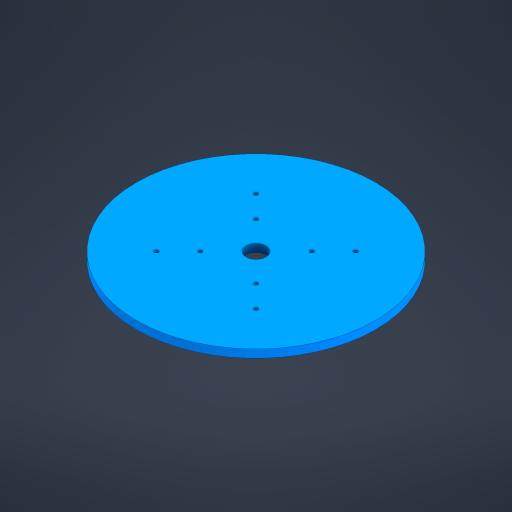
# Autodesk Inventor part: Foundation-Fork
Saved by Autodesk Inventor 2023 (Build 270158000, 158)
## iProperties
Created: 2023-09-02
Part Number: Foundation-Fork
Material: Generic
Document SubType Name: Modeling
Designer: Abhinav
Density: 1 g/cm^3
Appearance: Default(1)
Author: Abhinav
Autodesk Inventor part; units mm, degrees
ref_plane "YZ Plane" through (0, 0, 0) normal (1, 0, 0) x (0, 1, 0)
ref_plane "XZ Plane" through (0, 0, 0) normal (0, 1, 0) x (-1, 0, 0)
ref_plane "XY Plane" through (0, 0, 0) normal (0, 0, 1) x (1, 0, 0)
sketch "Sketch5" plane through (0, 0, -50) normal (0, -1, 0) x (1, 0, 0)
  line L0 (-90, 50) -> (35, 50) construction
  line L1 (60, 50) -> (-240, 50) construction
  line L2 (-180, 50) -> (0, 50) construction
  line L3 (0, 110) -> (0, -10) construction
  line L4 (-125, 85) -> (-55, 85) construction
  line L5 (-55, 85) -> (-55, 15) construction
  line L6 (-55, 15) -> (-125, 15) construction
  line L7 (-125, 15) -> (-125, 85) construction
  line L8 (-125, 85) -> (-55, 15) construction
  line L9 (-55, 85) -> (-125, 15) construction
  circle A0 centre (-90, 50) radius 150
  circle A1 centre (-125, 15) radius 2.5
  circle A2 centre (-55, 15) radius 2.5
  circle A3 centre (-55, 85) radius 2.5
  circle A4 centre (-125, 85) radius 2.5
  circle A5 centre (-90, 50) radius 12.5
  line L10 (-152.5, -12.5) -> (-27.5, -12.5) construction
  line L11 (-27.5, -12.5) -> (-27.5, 112.5) construction
  line L12 (-27.5, 112.5) -> (-152.5, 112.5) construction
  line L13 (-152.5, 112.5) -> (-152.5, -12.5) construction
  line L14 (-152.5, -12.5) -> (-27.5, 112.5) construction
  line L15 (-27.5, -12.5) -> (-152.5, 112.5) construction
  circle A6 centre (-152.5, -12.5) radius 2.5
  circle A7 centre (-27.5, -12.5) radius 2.5
  circle A8 centre (-27.5, 112.5) radius 2.5
  circle A9 centre (-152.5, 112.5) radius 2.5
  dimension "d57" = 300
  dimension "d25" = 125
  dimension "d50" = 70
  dimension "d51" = 70
  dimension "d52" = 5
  dimension "d53" = 25
  dimension "d54" = 125
  dimension "d55" = 125
  dimension "d56" = 5
  constraints: 30 end point, 10 coincident, 9 centre point, 6 equal radius, 4 horizontal, 4 midpoint, 4 parallel, 3 perpendicular, 1 horizontal alignment, 2 other
  measures "d25" distance of L0.start L0.end
  measures "d50" distance of L5.end L6.end
  measures "d51" distance of L4.end L5.end
  measures "d52" diameter of A1
  measures "d53" diameter of A5
  measures "d54" distance of L12.end L11.end
  measures "d55" distance of L11.end L10.end
  measures "d56" diameter of A6
extrude "Extrusion5" add sketch "Sketch5" along normal blind 10
body "Solid1"
